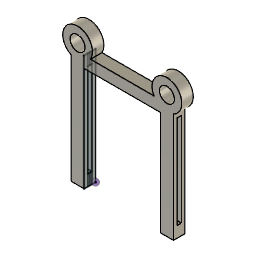
ajuste_1 (Autodesk Fusion 360 design; units mm, degrees)
part number: 2025-10-18-19-38-59-563
Autodesk Fusion 360 part; units mm, degrees
sketch "Sketch10" plane through (0, 0, 0) normal (1, 0, 0) x (0, 1, 0)
  line L0 (0, 0) -> (-3.1, 0)
  line L1 (-3.1, 0) -> (-3.1, 31)
  line L2 (-3.1, 31) -> (0, 31)
  line L3 (0, 31) -> (0, 0)
  line L4 (-1, 0) -> (-1, 31)
  line L5 (-2.1, 31) -> (-2.1, 0)
  line L6 (-2.1, 3) -> (-1, 3)
  line L7 (-1.55, 0) -> (-1.55, 3)
  line L8 (-2.1, 28) -> (-1, 28)
  line L9 (-1.55, 31) -> (-1.55, 28)
  dimension "d105" = 31
  dimension "d106" = 3.1
  dimension "d107" = 1.1
  dimension "d108" = 1
  dimension "d109" = 1
  dimension "d110" = 3
  dimension "d111" = 3
  constraint horizontal L0
  constraint vertical L1
  constraint horizontal L2
  constraint vertical L3
  constraint coincident L0.start L3.end
  constraint coincident L0 L4.start
  constraint coincident L2 L4.end
  constraint perpendicular L2 L4
  constraint coincident L2 L5.start
  constraint coincident L0 L5.end
  constraint perpendicular L0 L5
  constraint coincident L5 L6.start
  constraint coincident L4 L6.end
  constraint perpendicular L4 L6
  constraint midpoint L0 L7.start
  constraint midpoint L6 L7.end
  constraint coincident L5 L8.start
  constraint coincident L4 L8.end
  constraint perpendicular L4 L8
  constraint midpoint L2 L9.start
  constraint midpoint L8 L9.end
  measures "d105" distance of L0.start L2.end
  measures "d106" distance of L0.start L0.end
  measures "d107" distance of L4.start L5.end
  measures "d108" distance of L0.end L5.end
  measures "d109" distance of L0.start L4.start
  measures "d110" distance of L7.start L7.end
  measures "d111" distance of L9.start L9.end
sketch "Sketch11" plane through (0, 0, 0) normal (0, 1, 0) x (1, 0, 0)
  line L0 (0, 0, -3.1) -> (0, -31, -3.1)
  line L1 (0, -31) -> (0, 0)
  line L2 (0, -31, -3.1) -> (0, -31, 0)
  point P0 (0, -31)
  point P1 (0, -31)
  point P2 (0, -28)
  point P3 (0, -28)
  constraint coincident P1 P0
extrude "Extrude17" add sketch "Sketch10" along normal blind 3.5 contours L0 L2 L3 L4 | L0 L4 L6 L7 | L0 L5 L6 L7 | L2 L4 L8 L9 | L0 L1 L2 L5 | L2 L5 L8 L9 makes body 1
move_body "Move4" bodies 1 to x (1, 0, 0) y (0, 1, 0) z (0, 0, 1) at (20.5, 0, 0)
extrude "Extrude18" add sketch "Sketch10" against normal blind 3.5 separate body contours L0 L2 L3 L4 | L0 L4 L6 L7 | L0 L5 L6 L7 | L2 L4 L8 L9 | L0 L1 L2 L5 | L2 L5 L8 L9 makes body 2
sketch "Sketch13" plane through (0, 0, 0) normal (0, 1, 0) x (1, 0, 0)
  line L0 (20.5, -31, -3.1) -> (0, -31, -3.1)
  line L1 (20.5, -31) -> (0, -31)
  line L2 (20.5, -31, 0) -> (20.5, -31, -3.1)
  line L3 (0, -31, -3.1) -> (0, -31, 0)
  point P0 (20.5, -31)
  point P1 (0, -31)
  point P2 (20.5, -31)
  point P3 (0, -31)
  dimension "d134" = 20.5
  constraint coincident P2 P0
  constraint coincident P3 P1
  measures "d134" distance of P2 P1
extrude "Extrude19" add sketch "Sketch13" along normal blind 3 contours L0 L1 L2 L3 in plane through (0, 0, 31) normal (0, 0, -1) bodies 1 2
sketch "Sketch14" plane through (0, 0, 0) normal (0, 1, 0) x (1, 0, 0)
  line L0 (0, -28, -3.1) -> (-3.5, -28, -3.1)
  line L1 (-3.5, -28, -3.1) -> (-3.5, -31, -3.1)
  line L2 (-3.5, -31, -3.1) -> (0, -31, -3.1)
  line L3 (0, -31, -3.1) -> (0, -28, -3.1)
  line L4 (-3.5, -31, -3.1) -> (24, -31, -3.1)
  line L5 (-1.75, -31, -3.1) -> (-1.75, -28, -3.1)
  line L6 (-1.75, -28, -3.1) -> (-1.75, -33, -3.1)
  circle A0 through (0.25, -33, -3.1) (-2.75, -31.2679, -3.1) (-2.75, -34.7321, -3.1)
  circle A1 through (2.25, -33, -3.1) (-3.75, -29.5359, -3.1) (-3.75, -36.4641, -3.1)
  line L7 (24, -31, -3.1) -> (24, 0, -3.1)
  line L8 (20.5, -28, -3.1) -> (24, -28, -3.1)
  line L9 (24, -31, -3.1) -> (24, -28, -3.1)
  line L10 (20.5, -28, -3.1) -> (20.5, -31, -3.1)
  line L11 (22.25, -28, -3.1) -> (22.25, -31, -3.1)
  line L12 (20.5, -31, -3.1) -> (24, -31, -3.1)
  line L13 (22.25, -31, -3.1) -> (20.5, -31, -3.1)
  line L14 (22.25, -28, -3.1) -> (22.25, -33, -3.1)
  circle A2 through (24.25, -33, -3.1) (21.25, -31.2679, -3.1) (21.25, -34.7321, -3.1)
  circle A3 through (26.25, -33, -3.1) (20.25, -29.5359, -3.1) (20.25, -36.4641, -3.1)
  point P0 (0, -28)
  point P1 (-3.5, -31)
  point P2 (0, -31)
  point P3 (0, -28)
  point P4 (20.5, -28)
  dimension "d137" = 3.5
  dimension "d138" = 1.75
  dimension "d139" = 1.75
  dimension "d140" = 5
  dimension "d141" = 4
  dimension "d142" = 8
  dimension "d143" = 3.5
  dimension "d144" = 1.75
  dimension "d145" = 5
  dimension "d146" = 4
  dimension "d147" = 8
  constraint coincident P3 P0
  measures "d137" distance of P1 P2
extrude "Extrude20" add sketch "Sketch14" along normal blind 3.1 contours L3 L4 A1 | L2 L3 L4 L5 L6 A1 | L1 L2 L4 L5 L6 A1 | L1 L2 L4 A1 | L4 L10 L11 L12 L13 L14 A3 | L4 L7 L9 L12 L13 A3 | L4 L10 A3 | L4 L7 L9 L11 L12 L14 A3 in plane through (0, -3.1, 0) normal (0, 1, 0) bodies 1
other "Form1"
extrude "Extrude10" [suppressed]
move_body "Move2" [suppressed]
delete_body "RemoveBody1" bodies 3
sketch "Sketch8" plane through (0, 0, 0) normal (1, 0, 0) x (0, 1, 0)
  line L0 (3, 81) -> (21, 81)
  line L1 (0.4686, 78.5) -> (23.5, 78.5)
  line L2 (0.4686, 78.5) -> (0.4686, 83.5)
  line L3 (23.5, 83.5) -> (23.5, 78.5)
  line L4 (0.4686, 83.5) -> (23.5, 83.5)
  line L5 (23.5, 83.5) -> (23.5, 78.5)
  line L6 (23.5, 78.5) -> (0.4686, 78.5)
  line L7 (0.4686, 78.5) -> (0.4686, 83.5)
  line L8 (0.4686, 82.0062) -> (1.4686, 82.0062)
  line L9 (1.4686, 82.0062) -> (1.4686, 80.0062)
  line L10 (1.4686, 80.0062) -> (0.4686, 80.0062)
  line L11 (1.4686, 82.0062) -> (23.5, 82.0062)
  line L12 (0.4686, 80.0062) -> (23.5, 80.0062)
  line L13 (22.4687, 82.0062) -> (22.4687, 80.0062)
  line L14 (0.5, 56) -> (23.5, 56)
  line L15 (23.5, 56) -> (23.5, 53.5)
  line L16 (23.5, 53.5) -> (0.5, 53.5)
  line L17 (0.5, 53.5) -> (0.5, 56)
  line L18 (0.5, 58.5) -> (23.5, 58.5)
  line L19 (23.5, 58.5) -> (23.5, 56)
  line L20 (0.5, 56) -> (0.5, 58.5)
  line L21 (1.5, 56) -> (1.5, 57)
  line L22 (1.5, 56) -> (1.5, 55)
  line L23 (1.5, 55) -> (0.5, 55)
  line L24 (1.5, 57) -> (0.5, 57)
  line L25 (23.5, 57) -> (22.5, 57)
  line L26 (22.5, 56) -> (22.5, 57)
  line L27 (22.5, 56) -> (22.5, 55)
  line L28 (22.5, 55) -> (23.5, 55)
  dimension "d82" = 2
  dimension "d83" = 1
  dimension "d84" = 2
  constraint horizontal L0
  constraint horizontal L1
  constraint vertical L2
  constraint perpendicular L1 L3
  constraint horizontal L4
  constraint vertical L5
  constraint horizontal L6
  constraint vertical L7
  constraint coincident L2 L8.start
  constraint perpendicular L2 L8
  constraint perpendicular L8 L9
  constraint coincident L7 L10.end
  constraint perpendicular L7 L10
  constraint coincident L3 L11.end
  constraint perpendicular L3 L11
  constraint coincident L5 L12.end
  constraint perpendicular L5 L12
  constraint coincident L11 L13.start
  constraint coincident L12 L13.end
  constraint perpendicular L12 L13
  constraint horizontal L14
  constraint perpendicular L14 L15
  constraint perpendicular L15 L16
  constraint perpendicular L14 L17
  constraint perpendicular L15 L18
  constraint perpendicular L14 L19
  constraint perpendicular L18 L20
  constraint coincident L14 L21.start
  constraint perpendicular L14 L21
  constraint perpendicular L14 L22
  constraint coincident L17 L23.end
  constraint perpendicular L17 L23
  constraint coincident L20 L24.end
  constraint perpendicular L20 L24
  constraint coincident L19 L25.start
  constraint perpendicular L19 L25
  constraint coincident L14 L26.start
  constraint perpendicular L14 L27
  constraint coincident L15 L28.end
  constraint perpendicular L15 L28
  measures "d82" distance of L8.end L9.end
  measures "d83" distance of L8.start L8.end
  measures "d84" distance of L11.end L12.end
